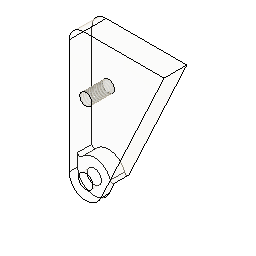
RampAngleLeft v3 (Autodesk Fusion 360 design; units mm, degrees)
Autodesk Fusion 360 part; units mm, degrees
sketch "Sketch1" plane through (0, 0, 0) normal (0, 1, 0) x (1, 0, 0)
  circle A0 centre (0, 0) radius 48 construction
  line L0 (0, 0) -> (0, 52) construction
  line L1 (0, 52) -> (-100, 52) construction
  line L2 (-9.746794, 47) -> (-100, 47) construction
  line L3 (-100, 47) -> (-100, 52) construction
  line L4 (-45.105246, -16.416967) -> (-39.632924, -31.452049) construction
  line L5 (0, 0) -> (-48, 0) construction
  line L6 (-45.105246, -16.416967) -> (0, 0) construction
  line L7 (-43.502774, -20.285677) -> (-36.740882, -34.786601) construction
  line L8 (-43.502774, -20.285677) -> (0, 0) construction
  line L9 (0, 52) -> (100, 52) construction
  line L10 (100, 52) -> (100, 32) construction
  circle A1 centre (100, 32) radius 20 construction
  line L11 (86.5, 46.756355) -> (113.5, 46.756355) construction
  line L12 (86.5, 46.756355) -> (100, 12) construction
  line L13 (113.5, 46.756355) -> (100, 12) construction
  line L14 (100, 32) -> (100, 12) construction
  line L15 (91.3, 50.008609) -> (108.7, 50.008609) construction
  line L16 (91.3, 50.008609) -> (100, 12) construction
  line L17 (108.7, 50.008609) -> (100, 12) construction
  circle A2 centre (0, 0) radius 14 construction
  circle A3 centre (-31.949549, -11.628685) radius 20 construction
  circle A4 centre (-30.814465, -14.369021) radius 20 construction
  line L18 (-45.105246, -16.416967) -> (-50.743402, -18.469088) construction
  line L19 (-43.502774, -20.285677) -> (-48.94062, -22.821386) construction
  line L20 (-53.694035, -7.895252) -> (-40.366113, -36.477074)
  line L21 (-40.366113, -36.477074) -> (-57.366113, -36.477074)
  line L22 (-60.366113, -33.477074) -> (-60.366113, -9.374416)
  arc A5 (-53.694035, -7.895252) -> (-60.366113, -9.374416) centre (-56.866113, -9.374416) ccw
  arc A6 (-60.366113, -9.374416) -> (-53.694035, -7.895252) centre (-56.866113, -9.374416) ccw
  arc A7 (-60.366113, -33.477074) -> (-57.366113, -36.477074) centre (-57.366113, -33.477074) ccw
  circle A8 centre (-56.866113, -9.374416) radius 1.5
  line L23 (-56.866113, -9.374416) -> (-56.866113, -24.374416) construction
  circle A9 centre (-56.866113, -24.374416) radius 1.5
  line L24 (-53.577189, -8.177345) -> (-43.27693, -36.477074) construction
  line L25 (-60.352794, -9.06937) -> (-62.750658, -36.477074) construction
  line L26 (-62.750658, -36.477074) -> (-60.366113, -36.477074) construction
  line L27 (-60.366113, -36.477074) -> (-57.366113, -36.477074) construction
  line L28 (-56.866113, -9.374416) -> (-58.173449, -24.317336) construction
  arc A10 (-58.173449, -24.317336) -> (-56.866113, -24.374416) centre (-56.866113, -9.374416) ccw construction
  circle A11 centre (-58.173449, -24.317336) radius 1.5 construction
  line L29 (-58.173449, -24.317336) -> (-58.304182, -25.811628) construction
  line L30 (-56.866113, -24.374416) -> (-56.866113, -25.874416) construction
  arc A12 (-58.042715, -22.823044) -> (-56.866113, -22.874416) centre (-56.866113, -9.374416) ccw construction
  arc A13 (-58.304182, -25.811628) -> (-56.866113, -25.874416) centre (-56.866113, -9.374416) ccw construction
  point P0 (100, 46.756355)
  point P1 (-47.128005, -21.97615)
  point P2 (-45.105246, -16.416967)
  point P3 (-13.155697, -4.788282)
  point P4 (-12.688309, -5.916656)
  point P5 (-60.366113, -36.477074)
  point P6 (-58.042715, -22.823044)
  point P7 (-56.866113, -22.874416)
  point P8 (-56.866113, -25.874416)
  point P9 (-58.304182, -25.811628)
  dimension "d1" = 96
  dimension "d2" = 52
  dimension "d3" = 100
  dimension "d4" = 5
  dimension "d5" = 16
  dimension "d6" = 70
  dimension "d7" = 16
  dimension "d8" = 65
  dimension "d9" = 100
  dimension "d10" = 20
  dimension "d11" = 27
  dimension "d12" = 40
  dimension "d13" = 4.8
  dimension "d16" = 17.4
  dimension "d17" = 38.008609
  dimension "d18" = 34.756355
  dimension "d20" = 28
  dimension "d21" = 40
  dimension "d22" = 40
  dimension "d23" = 34
  dimension "d24" = 38
  dimension "d25" = 4
  dimension "d26" = 21.97615
  dimension "d29" = 16
  dimension "d30" = 20
  dimension "d31" = 7
  dimension "d32" = 3
  dimension "d35" = 3
  dimension "d36" = 15
  dimension "d37" = 3
  dimension "d38" = 5
  dimension "d39" = 5
  dimension "d40" = 3
  dimension "d41" = 13.5
  dimension "d42" = 16.5
  dimension "d43" = 3.5
  dimension "d44" = 56.866113
  dimension "d45" = 9.374416
  constraint coincident A0.centre L0.start
  constraint vertical L0
  constraint perpendicular L0 L1
  constraint parallel L1 L2
  constraint perpendicular L1 L3
  constraint tangent A0 L4
  constraint coincident A0 L5.end
  constraint perpendicular L0 L5
  constraint tangent A0 L7
  constraint perpendicular L0 L9
  constraint perpendicular L9 L10
  constraint coincident L10.end A1.centre
  constraint coincident L9.end A1
  constraint perpendicular L10 L11
  constraint coincident A1 L12.end
  constraint vertical L14
  constraint parallel L11 L15
  constraint concentric A0 A2
  constraint tangent A2 A3
  constraint tangent A2 A4
  constraint perpendicular L4 L18
  constraint perpendicular L7 L19
  constraint parallel L7 L20
  constraint horizontal L21
  constraint perpendicular L21 L22
  constraint tangent L20 A5
  constraint tangent L22 A5
  constraint concentric A5 A6
  constraint tangent L22 A7
  constraint tangent L21 A7
  constraint concentric A5 A8
  constraint vertical L23
  constraint parallel L4 L24
  constraint tangent A6 L24
  constraint parallel L21 L26
  constraint parallel L23 L30
  constraint collinear L28 L29
  constraint tangent A5 L25
  measures "d1" diameter of A0
  measures "d2" distance of A0.centre L0.end
  measures "d3" distance of L0.end L1.end
  measures "d4" distance of L1 L2
  measures "d6" angle of L4 L5
  measures "d8" angle of L5 L7
  measures "d9" distance of L0.end L9.end
  measures "d10" distance of L9.end L10.end
  measures "d12" diameter of A1
  measures "d17" distance of L12.end L15
  measures "d18" distance of L11 L12.end
  measures "d20" diameter of A2
  measures "d21" diameter of A3
  measures "d22" diameter of A4
  measures "d31" diameter of A5
  measures "d32" radius of A7
  measures "d35" diameter of A8
  measures "d37" diameter of A9
  measures "d38" angle of L22 L25
  measures "d39" angle of L23 L28
  measures "d40" diameter of A11
  measures "d41" radius of A12
  measures "d42" radius of A13
extrude "Extrude1" add sketch "Sketch1" along normal blind 4.8
thread "Thread1" "ISO Metric profile 3.0 M3x0.5 6H" major diameter 3.086 minor diameter 2.529 pitch 0.5 angle 60 resizes the face on face at (-57.858641, 3.2, 25.499087)
sketch "Sketch2" plane through (0, 4.8, 0) normal (0, 1, 0) x (-1, 0, 0)
  arc A0 (53.694035, 7.895252) -> (60.366113, 9.374416) centre (56.866113, 9.374416) ccw
  line L0 (60.366113, 9.374416) -> (60.366113, 33.477074)
  arc A1 (60.366113, 33.477074) -> (57.366113, 36.477074) centre (57.366113, 33.477074) ccw
  line L1 (57.366113, 36.477074) -> (40.366113, 36.477074)
  line L2 (40.366113, 36.477074) -> (53.694035, 7.895252)
  circle A2 centre (56.866113, 9.374416) radius 1.5
  arc A3 (60.366113, 9.374416) -> (53.694035, 7.895252) centre (56.866113, 9.374416) ccw
  circle A4 centre (56.866113, 24.374416) radius 1.2645
extrude "Extrude3" cut sketch "Sketch2" against normal blind 3 contours A0 A3 picked at (54.212104, 8.403446)
fillet "Fillet2" radius 0.5 2 edges at (-60.366113, 3.3, 9.374416) (-53.694035, 3.3, 7.895252)
